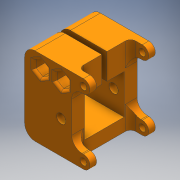
# Autodesk Inventor part: arm_socket
Saved by Autodesk Inventor 2016 (Build 200138000, 138)
## iProperties
Created: 2016-10-27
Part Number: arm_socket
Material: Generic
Document SubType Name: Modeling
Designer: Jakub
Density: 1 g/cm^3
Appearance: Default
Author: Jakub
Autodesk Inventor part; units mm, degrees
ref_plane "YZ Plane" through (0, 0, 0) normal (1, 0, 0) x (0, 1, 0)
ref_plane "XZ Plane" through (0, 0, 0) normal (0, 1, 0) x (-1, 0, 0)
ref_plane "XY Plane" through (0, 0, 0) normal (0, 0, 1) x (1, 0, 0)
sketch "Sketch1" plane through (0, 0, 0) normal (1, 0, 0) x (0, 1, 0)
  line L0 (-12.5, 15) -> (12.5, 15)
  line L1 (12.5, 15) -> (12.5, -15)
  line L2 (12.5, -15) -> (-12.5, -15)
  line L3 (-12.5, -15) -> (-12.5, 15)
  line L4 (-12.5, 15) -> (12.5, -15) construction
  line L5 (12.5, 15) -> (-12.5, -15) construction
  line L6 (-7.55, 5.1) -> (7.55, 5.1)
  line L7 (7.55, 5.1) -> (7.55, -10)
  line L8 (7.55, -10) -> (-7.55, -10)
  line L9 (-7.55, -10) -> (-7.55, 5.1)
  line L10 (-7.55, 5.1) -> (7.55, -10) construction
  line L11 (7.55, 5.1) -> (-7.55, -10) construction
  line L12 (0, 5.1) -> (1, 5.1)
  line L13 (1, 5.1) -> (-1, 5.1)
  line L14 (-1, 5.1) -> (-1, 15)
  line L15 (-1, 15) -> (1, 15)
  line L16 (1, 15) -> (1, 5.1)
  point P0 (0, 0)
  point P1 (0, -2.45)
  dimension "d0" = 25
  dimension "d1" = 30
  dimension "d2" = 15.1
  dimension "d3" = 15.1
  dimension "d4" = 5
  dimension "d5" = 4.95
  dimension "d6" = 1
  dimension "d7" = 2
  constraints: 34 end point, 6 parallel, 5 midpoint, 3 horizontal, 3 perpendicular, 2 point on line
  measures "d0" distance of L1.end L2.end
  measures "d1" distance of L0.end L1.end
  measures "d2" distance of L7.end L8.end
  measures "d3" distance of L6.end L7.end
  measures "d4" distance between parallel lines of L2 L8
  measures "d5" distance between parallel lines of L1 L7
  measures "d6" distance of L12.start L12.end
  measures "d7" distance of L14.end L15.end
extrude "Extrusion1" add sketch "Sketch1" along normal blind 8 contours L0 L14 L6 L9 L8 L7 L16 L1 L2 L3
sketch "Sketch2" plane through (0, 12.5, 15) normal (0, 1, 0) x (1, 0, 0)
  line L0 (0, 0) -> (8, 0) projected
  line L1 (4, 0) -> (4, 5)
  circle A0 centre (4, 5) radius 1.25
  point P0 (0, 15)
  dimension "d10" = 5
  dimension "d11" = 2.5
  constraints: 2 end point, 1 centre point, 1 coincident, 1 midpoint, 1 vertical
  measures "d10" distance of L1.start L1.end
  measures "d11" diameter of A0
extrude "Extrusion2" cut sketch "Sketch2" against normal through all
sketch "Sketch3" plane through (0, 12.5, 15) normal (0, 1, 0) x (1, 0, 0)
  line L0 (0, 30) -> (8, 30) projected
  line L1 (4, 30) -> (4, 17.45)
  circle A0 centre (4, 17.45) radius 1.75
  point P0 (0, 15)
  dimension "d14" = 12.55
  dimension "d15" = 3.5
  constraints: 2 end point, 1 centre point, 1 coincident, 1 midpoint, 1 vertical
  measures "d14" distance of L1.start L1.end
  measures "d15" diameter of A0
extrude "Extrusion3" cut sketch "Sketch3" against normal through all
sketch "Sketch4" plane through (0, 12.5, 15) normal (0, 1, 0) x (1, 0, 0)
  circle A0 centre (4, 5) radius 1.25 projected
  circle A1 centre (4, 5) radius 2.5
  point P0 (0, 15)
  dimension "d18" = 5
  constraints: 1 centre point, 1 coincident
  measures "d18" diameter of A1
extrude "Extrusion4" cut sketch "Sketch4" against normal blind 5
sketch "Sketch5" plane through (0, -12.5, -15) normal (0, -1, 0) x (1, 0, 0)
  circle A0 centre (4, 25) radius 1.25 projected
  line L0 (4, 28) -> (6.5981, 26.5)
  line L1 (6.5981, 26.5) -> (6.5981, 23.5)
  line L2 (6.5981, 23.5) -> (4, 22)
  line L3 (4, 22) -> (1.4019, 23.5)
  line L4 (1.4019, 23.5) -> (1.4019, 26.5)
  line L5 (1.4019, 26.5) -> (4, 28)
  point P0 (0, 15)
  dimension "d21" = 3
  constraints: 12 end point, 1 coincident, 13 other
  measures "d21" distance of L3.end L4.end
extrude "Extrusion5" cut sketch "Sketch5" against normal blind 5
fillet "Fillet1" radius 1 1 edges at (1.5, 12.5, 10)
fillet "Fillet2" radius 1 6 edges at (2.701, -12.5, 12.25) (5.299, -12.5, 12.25) (6.5981, -12.5, 10) (5.299, -12.5, 7.75) (2.701, -12.5, 7.75) (1.4019, -12.5, 10)
sketch "Sketch6" plane through (8, 0, 0) normal (1, 0, 0) x (0, 0, -1)
  line L0 (15, 12.5) -> (-15, 12.5) projected
  line L1 (-15, 12.5) -> (-10, 12.5)
  line L2 (-10, 12.5) -> (-10, 10)
  line L3 (-10, 10) -> (-15, 10)
  line L4 (-15, 10) -> (-15, 12.5)
  line L5 (15, 12.5) -> (10, 12.5)
  line L6 (10, 12.5) -> (10, 10)
  line L7 (10, 10) -> (15, 10)
  line L8 (15, 10) -> (15, 12.5)
  line L9 (-15, -12.5) -> (15, -12.5) projected
  line L10 (-15, -12.5) -> (-10, -12.5)
  line L11 (-10, -12.5) -> (-10, -10)
  line L12 (-10, -10) -> (-15, -10)
  line L13 (-15, -10) -> (-15, -12.5)
  line L14 (15, -12.5) -> (10, -12.5)
  line L15 (10, -12.5) -> (10, -10)
  line L16 (10, -10) -> (15, -10)
  line L17 (15, -10) -> (15, -12.5)
  point P0 (0, 0)
  dimension "d26" = 5
  dimension "d27" = 2.5
  dimension "d28" = 5
  dimension "d29" = 2.5
  dimension "d30" = 5
  dimension "d31" = 2.5
  dimension "d32" = 5
  dimension "d33" = 2.5
  constraints: 32 end point, 8 parallel, 4 horizontal, 4 perpendicular
  measures "d26" distance of L2.end L3.end
  measures "d27" distance of L1.end L2.end
  measures "d28" distance of L7.end L6.end
  measures "d29" distance of L6.end L5.end
  measures "d30" distance of L12.end L11.end
  measures "d31" distance of L11.end L10.end
  measures "d32" distance of L15.end L16.end
  measures "d33" distance of L14.end L15.end
extrude "Extrusion6" add sketch "Sketch6" along normal blind 7
fillet "Fillet3" radius 2.5 8 edges at (15, 11.25, 15) (15, 11.25, 10) (15, -11.25, 15) (15, -11.25, 10) (15, -11.25, -10) (15, -11.25, -15) (15, 11.25, -10) (15, 11.25, -15)
sketch "Sketch7" plane through (0, -12.5, -15) normal (0, -1, 0) x (1, 0, 0)
  arc A0 (12.5, 25) -> (12.5, 30) centre (12.5, 27.5) ccw projected
  circle A1 centre (12.5, 27.5) radius 1.25
  arc A2 (12.5, 0) -> (12.5, 5) centre (12.5, 2.5) ccw projected
  circle A3 centre (12.5, 2.5) radius 1.25
  point P0 (0, 15)
  dimension "d37" = 2.5
  dimension "d38" = 2.5
  constraints: 2 centre point, 2 coincident
  measures "d37" diameter of A1
  measures "d38" diameter of A3
extrude "Extrusion7" cut sketch "Sketch7" against normal through all
fillet "Fillet4" radius 2 4 edges at (8, -10, 12.5) (8, 10, 12.5) (8, 10, -12.5) (8, -10, -12.5)
fillet "Fillet5" radius 4 4 edges at (8, -11.25, 10) (8, -11.25, -10) (8, 11.25, -10) (8, 11.25, 10)
sketch "Sketch8" plane through (0, 0, 0) normal (-1, 0, 0) x (0, 0, 1)
  line L0 (5.1, 1) -> (5.1, 7.55) projected
  line L1 (5.1, 1) -> (5.1, 7.55)
  line L2 (-10, 7.55) -> (5.1, 7.55) projected
  line L3 (5.1, 7.55) -> (-10, 7.55)
  line L4 (-10, -7.55) -> (-10, 7.55) projected
  line L5 (-10, 7.55) -> (-10, -7.55)
  line L6 (5.1, -7.55) -> (-10, -7.55) projected
  line L7 (-10, -7.55) -> (5.1, -7.55)
  line L8 (5.1, -1) -> (5.1, -7.55) projected
  line L9 (5.1, -7.55) -> (5.1, -1)
  line L10 (15, -1) -> (15, -12.5) projected
  line L11 (5.1, -1) -> (15, -1)
  line L12 (15, -1) -> (15, -12.5)
  line L13 (15, -12.5) -> (-15, -12.5) projected
  line L14 (15, -12.5) -> (-15, -12.5)
  line L15 (-15, -12.5) -> (-15, 12.5) projected
  line L16 (-15, -12.5) -> (-15, 12.5)
  line L17 (10, 12.5) -> (15, 12.5) projected
  line L18 (-15, 12.5) -> (15, 12.5)
  line L19 (15, 8) -> (15, 1) projected
  line L20 (15, 12.5) -> (15, 1)
  line L21 (15, 1) -> (5.1, 1)
  point P0 (0, 0)
  constraints: 24 end point, 7 collinear, 5 perpendicular
extrude "Extrusion8" add sketch "Sketch8" along normal blind 10
fillet "Fillet7" radius 4 3 edges at (-10, 6.75, 15) (-10, -6.75, 15) (-10, 0, -15)
pattern_linear "Rectangular Pattern1" count 2 spacing 8 along (-1, 0, 0) of "Extrusion2", "Extrusion5", "Fillet2", "Extrusion4", "Fillet1"
equation "\"d19\" = d18"
body "Solid1"
